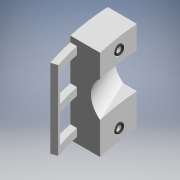
# Autodesk Inventor part: 8099429 CMMT-AS-C7/C12-11A-P3---(clamp)
Saved by Autodesk Inventor 2017.3 (Build 213256000, 256)
## iProperties
Part Number: 8099429 CMMT-AS-C7/C12-11A-P3---(clamp)
Material: Generic
Catalog Web Link: www.cadenas.de
Description: CMMT-clamp-Shield clamp
Vendor: FESTO
Document SubType Name: Modeling
Designer: partserver
Manufacturer: FESTO
Mass: 26.8019 g
Surface Area: 87.6316 cm^2
Volume: 26.8019 cm^3
Density: 1 g/cm^3
Appearance: PSOLRGB-255-255-255
Category: PARTsolutions
Company: FESTO
Title: 8099429 CMMT-AS-C7/C12-11A-P3---(clamp)
Author: Cadenas PARTsolutions
Comments: Shield clamp
PSOL_IDENT_0: {$CADENAS_DATA\23d-libs\festo\parts\c\cmmt\parts\cmmt_clamp.prj},222 {VTYP=3D},{NB=8099429 CMMT-AS-C
PSOL_IDENT_1: 7/C12-11A-P3---(clamp)},{LINA=8099429 CMMT-AS-C7/C12-11A-P3---(clamp)},{NN=CMMT-clamp},{DATE=07.10.2
PSOL_IDENT_2: 020 06:56:02},{GEOMDATE=07.10.2020 06:45:00},{VERSION=},{LINEID=30},{WBVAR=},{WBNUMERIC=}  {NB=80994
PSOL_IDENT_3: 29 CMMT-AS-C7/C12-11A-P3---(clamp)},{LINA=8099429 CMMT-AS-C7/C12-11A-P3---(clamp)},{KT=DUMMY},{TNR=8
PSOL_IDENT_4: 099429},{TYP=CMMT-AS-C7/C12-11A-P3},{B1=58.500},{B2=18.000},{B3=44.000},{H1=46.200},{H2=28.200},{R1=
PSOL_IDENT_5: 181.500},{B4=23.350},{H3=13.100}
NB: 8099429 CMMT-AS-C7/C12-11A-P3---(clamp)
NN: CMMT-clamp
NT: Shield clamp
NBSYN: $TNR. $TYP.---(clamp)
LINA: 8099429 CMMT-AS-C7/C12-11A-P3---(clamp)
CATALOG: Festo
TNR: 8099429
TYP: CMMT-AS-C7/C12-11A-P3
B1: 58.5
B2: 18
B3: 44
H1: 46.2
H2: 28.2
R1: 181.5
B4: 23.35
H3: 13.1
SUPPLIER: FESTO
ARTICLENO: 8099429 CMMT-AS-C7/C12-11A-P3---(clamp)
BOMINFO: 8099429 CMMT-AS-C7/C12-11A-P3---(clamp)
CREATOR: CADENAS GmbH
Autodesk Inventor part; units mm, degrees
sketch "Sketch_12" plane through (0, 0, 0) normal (0, 0, 1) x (1, 0, 0)
  arc A0 (-4.225, -27.8912) -> (-3.982, -28.2) centre (-3.982, -27.95) ccw
  line L0 (-3.982, -28.2) -> (10.808, -28.2)
  arc A1 (6.2129, -44.6526) -> (10.808, -28.2) centre (-156.3668, 9.6224) ccw
  arc A2 (6.2129, -44.6526) -> (6.3707, -44.9689) centre (6.4501, -44.7318) ccw
  line L1 (6.3707, -44.9689) -> (10.0502, -46.2)
  arc A3 (10.0502, -46.2) -> (19.016, -0.5326) centre (-162.0972, 11.311) ccw
  arc A4 (19.016, -0.5326) -> (18.517, 0) centre (18.517, -0.5) ccw
  line L2 (18.517, 0) -> (0.2345, 0)
  arc A5 (0.2345, 0) -> (-0.015, -0.2338) centre (0.2345, -0.25) ccw
  arc A6 (-4.225, -27.8912) -> (-0.015, -0.2338) centre (-162.1732, 10.3007) ccw
  constraints: 14 point on circle, 7 centre point, 6 end point
extrude "Extrusion1" add sketch "Sketch_12" along normal mid plane 58.5
sketch "Sketch_2" plane through (0, 0, 0) normal (1, 0, 0) x (0, 1, 0)
  line L0 (-28.4, 20.5) -> (-43, 20.5)
  arc A0 (-43, 20.5) -> (-43.2, 20.3) centre (-43, 20.3) ccw
  line L1 (-43.2, 20.3) -> (-43.2, 2.7)
  arc A1 (-43.2, 2.7) -> (-43, 2.5) centre (-43, 2.7) ccw
  line L2 (-43, 2.5) -> (-28.4, 2.5)
  arc A2 (-28.4, 2.5) -> (-28.2, 2.7) centre (-28.4, 2.7) ccw
  line L3 (-28.2, 2.7) -> (-28.2, 20.3)
  arc A3 (-28.2, 20.3) -> (-28.4, 20.5) centre (-28.4, 20.3) ccw
  constraints: 8 end point, 8 point on circle, 4 centre point
extrude "Extrusion2" cut sketch "Sketch_2" along normal blind 15
sketch "Sketch_3" plane through (0, 0, 0) normal (1, 0, 0) x (0, 1, 0)
  arc A0 (-43, -2.5) -> (-43.2, -2.7) centre (-43, -2.7) ccw
  line L0 (-43.2, -2.7) -> (-43.2, -20.3)
  arc A1 (-43.2, -20.3) -> (-43, -20.5) centre (-43, -20.3) ccw
  line L1 (-43, -20.5) -> (-28.4, -20.5)
  arc A2 (-28.4, -20.5) -> (-28.2, -20.3) centre (-28.4, -20.3) ccw
  line L2 (-28.2, -20.3) -> (-28.2, -2.7)
  arc A3 (-28.2, -2.7) -> (-28.4, -2.5) centre (-28.4, -2.7) ccw
  line L3 (-28.4, -2.5) -> (-43, -2.5)
  constraints: 8 end point, 8 point on circle, 4 centre point
extrude "Extrusion3" cut sketch "Sketch_3" along normal blind 15
sketch "Sketch_4" plane through (13.01, 0, 0) normal (1, 0, 0) x (0, 0, -1)
  line L0 (-29.25, -48.1) -> (-25.5, -48.1)
  line L1 (-25.5, -48.1) -> (-25.5, -28.2)
  line L2 (-25.5, -28.2) -> (-29.25, -28.2)
  line L3 (-29.25, -28.2) -> (-29.25, -48.1)
  constraints: 8 end point
extrude "Extrusion4" cut sketch "Sketch_4" along normal mid plane 40
sketch "Sketch_5" plane through (13.01, 0, 0) normal (1, 0, 0) x (0, 0, -1)
  line L0 (25.5, -48.1) -> (29.25, -48.1)
  line L1 (29.25, -48.1) -> (29.25, -28.2)
  line L2 (29.25, -28.2) -> (25.5, -28.2)
  line L3 (25.5, -28.2) -> (25.5, -48.1)
  constraints: 8 end point
extrude "Extrusion5" cut sketch "Sketch_5" along normal mid plane 30
sketch "Sketch_6" plane through (0, -13.1, 0) normal (0, 1, 0) x (1, 0, 0)
  line L0 (-3, -22) -> (21.09, -22)
  line L1 (21.09, -22) -> (21.09, -26)
  line L2 (21.09, -26) -> (14.34, -26)
  arc A0 (14.09, -25.75) -> (14.34, -26) centre (14.34, -25.75) ccw
  line L3 (14.09, -25.75) -> (14.09, -24.25)
  line L4 (14.09, -24.25) -> (-0.91, -24.7738)
  line L5 (-0.91, -24.7738) -> (-0.91, -25.5)
  line L6 (-0.91, -25.5) -> (-3, -25.5)
  line L7 (-3, -25.5) -> (-3, -22)
  line L8 (-3, -22) -> (21.09, -22)
  constraints: 18 end point, 2 point on circle, 1 centre point
revolve "Revolution1" cut sketch "Sketch_6" angle 360 about axis through (-3, -13.1, 22) along (-1, 0, 0)
sketch "Sketch_7" plane through (0, -13.1, 0) normal (0, 1, 0) x (1, 0, 0)
  line L0 (-3, 22) -> (21.09, 22)
  line L1 (21.09, 22) -> (21.09, 18)
  line L2 (21.09, 18) -> (14.34, 18)
  arc A0 (14.09, 18.25) -> (14.34, 18) centre (14.34, 18.25) ccw
  line L3 (14.09, 18.25) -> (14.09, 19.75)
  line L4 (14.09, 19.75) -> (-0.91, 19.2262)
  line L5 (-0.91, 19.2262) -> (-0.91, 18.5)
  line L6 (-0.91, 18.5) -> (-3, 18.5)
  line L7 (-3, 18.5) -> (-3, 22)
  line L8 (-3, 22) -> (21.09, 22)
  constraints: 18 end point, 2 point on circle, 1 centre point
revolve "Revolution2" cut sketch "Sketch_7" angle 360 about axis through (-3, -13.1, -22) along (-1, 0, 0)
sketch "Sketch_8" plane through (0, -13.1, 0) normal (0, 1, 0) x (1, 0, 0)
  line L0 (-2, -22) -> (-0.75, -22)
  circle A0 centre (-1.375, -24.5) radius 0.625
  constraints: 2 end point, 1 centre point
revolve "Revolution3" add sketch "Sketch_8" angle 360 about axis through (-2, -13.1, 22) along (-1, 0, 0)
sketch "Sketch_13" plane through (0, -13.1, 0) normal (0, 1, 0) x (1, 0, 0)
  line L0 (-2, 22) -> (-0.75, 22)
  circle A0 centre (-1.375, 19.5) radius 0.625
  constraints: 2 end point, 1 centre point
revolve "Revolution4" add sketch "Sketch_13" angle 360 about axis through (-2, -13.1, -22) along (-1, 0, 0)
sketch "Sketch_10" plane through (0, -27.2, 0) normal (0.4226, 0.9063, 0) x (0.9063, -0.4226, 0)
  line L0 (-16.5, -8.5) -> (-3.428, -8.5)
  arc A0 (-3.428, -8.5) -> (-3.428, 14.5) centre (-13.0587, 3) ccw
  line L1 (-3.428, 14.5) -> (-16.5, 14.5)
  line L2 (-16.5, 14.5) -> (-16.5, -8.5)
  constraints: 6 end point, 2 point on circle, 1 centre point
extrude "Extrusion6" cut sketch "Sketch_10" along normal mid plane 70
ref_plane "ANBAU_XY" through (0, 0, 0) normal (1, 0, 0) x (0, 0, -1)
ref_plane "ANBAU_YZ" through (0, 0, 0) normal (0, 0, -1) x (0, 1, 0)
ref_plane "ANBAU_ZX" through (0, 0, 0) normal (0, 1, 0) x (1, 0, 0)
ref_plane "SCREW_1_XY" through (14.09, -13.1, 22) normal (1, 0, 0) x (0, 0, -1)
ref_plane "SCREW_1_YZ" through (14.09, -13.1, 22) normal (0, 0, -1) x (0, 1, 0)
ref_plane "SCREW_1_ZX" through (14.09, -13.1, 22) normal (0, 1, 0) x (1, 0, 0)
ref_plane "SCREW_2_XY" through (14.09, -13.1, -22) normal (1, 0, 0) x (0, 0, -1)
ref_plane "SCREW_2_YZ" through (14.09, -13.1, -22) normal (0, 0, -1) x (0, 1, 0)
ref_plane "SCREW_2_ZX" through (14.09, -13.1, -22) normal (0, 1, 0) x (1, 0, 0)
body "Solid1"
